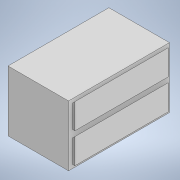
# Autodesk Inventor part: drawer
Saved by Autodesk Inventor 2022 (Build 260153000, 153)
## iProperties
Created: 2022-05-13
Part Number: drawer
Material: Generic
Document SubType Name: Modeling
Designer: compsci
Density: 1 g/cm^3
Appearance: Default
Author: compsci
Autodesk Inventor part; units mm, degrees
ref_plane "YZ Plane" through (0, 0, 0) normal (1, 0, 0) x (0, 1, 0)
ref_plane "XZ Plane" through (0, 0, 0) normal (0, 1, 0) x (-1, 0, 0)
ref_plane "XY Plane" through (0, 0, 0) normal (0, 0, 1) x (1, 0, 0)
sketch "Sketch2" plane through (0, 0, 0) normal (0, 1, 0) x (-1, 0, 0)
  line L0 (-304.8, 508) -> (304.8, 508)
  line L1 (304.8, 508) -> (304.8, -508)
  line L2 (304.8, -508) -> (-304.8, -508)
  line L3 (-304.8, -508) -> (-304.8, 508)
  line L4 (-304.8, 508) -> (304.8, -508) construction
  line L5 (304.8, 508) -> (-304.8, -508) construction
  point P0 (0, 0)
  dimension "d2" = 609.6
  dimension "d3" = 1016
  constraints: 12 end point, 2 midpoint, 2 parallel, 1 horizontal, 1 perpendicular
  measures "d2" distance of L0.start L0.end
  measures "d3" distance of L2.end L0.start
extrude "Extrusion1" add sketch "Sketch2" along normal blind 609.6
sketch "Sketch3" plane through (304.8, 0, 508) normal (1, 0, 0) x (0, 0, -1)
  line L0 (0, 0) -> (1016, 0) projected
  line L1 (1016, 0) -> (1016, 609.6) projected
  line L2 (0, 609.6) -> (1016, 609.6) projected
  line L3 (0, 0) -> (0, 609.6) projected
  line L4 (0, 0) -> (0, 609.6) projected
  line L5 (1016, 0) -> (1016, 609.6) projected
  line L6 (1016, 0) -> (0, 0) projected
  line L7 (0, 304.8) -> (1016, 304.8)
  line L8 (1016, 304.8) -> (1016, 0)
  line L9 (1016, 0) -> (0, 0)
  line L10 (0, 0) -> (0, 304.8)
  line L11 (0, 304.8) -> (1016, 304.8)
  line L12 (1016, 304.8) -> (1016, 609.6)
  line L13 (1016, 609.6) -> (0, 609.6)
  line L14 (0, 609.6) -> (0, 304.8)
  line L15 (977.9, 266.7) -> (38.1, 266.7)
  line L16 (38.1, 266.7) -> (38.1, 38.1)
  line L17 (38.1, 38.1) -> (977.9, 38.1)
  line L18 (977.9, 38.1) -> (977.9, 266.7)
  line L19 (977.9, 342.9) -> (38.1, 342.9)
  line L20 (38.1, 342.9) -> (38.1, 571.5)
  line L21 (38.1, 571.5) -> (977.9, 571.5)
  line L22 (977.9, 571.5) -> (977.9, 342.9)
  point P0 (508, 0)
  dimension "d5" = 38.1
  dimension "d6" = 38.1
  constraints: 32 end point, 8 parallel, 4 perpendicular, 2 horizontal, 1 midpoint, 6 other
  measures "d5" distance between parallel lines of L7 L15
  measures "d6" distance between parallel lines of L11 L19
extrude "Extrusion2" add sketch "Sketch3" along normal blind 25.4 contours L18 L17 L16 L15 | L19 L20 L21 L22
sketch "Sketch4" plane through (304.8, 38.1, 469.9) normal (0, 0, 1) x (1, 0, 0)
  line L0 (0, 304.8) -> (0, 533.4) projected
  line L1 (0, 304.8) -> (25.4, 304.8) projected
  line L2 (25.4, 533.4) -> (25.4, 304.8) projected
  line L3 (0, 533.4) -> (25.4, 533.4) projected
  line L4 (0, 0) -> (0, 228.6) projected
  line L5 (0, 0) -> (25.4, 0) projected
  line L6 (25.4, 228.6) -> (25.4, 0) projected
  line L7 (0, 228.6) -> (25.4, 228.6) projected
  line L8 (25.4, 228.6) -> (25.4, 0) projected
  line L9 (25.4, 228.6) -> (25.4, 254)
  line L10 (0, 228.6) -> (25.4, 228.6) projected
  line L11 (25.4, 254) -> (0, 228.6)
  line L12 (25.4, 533.4) -> (25.4, 304.8) projected
  line L13 (25.4, 533.4) -> (25.4, 558.8)
  line L14 (0, 533.4) -> (25.4, 533.4) projected
  line L15 (25.4, 558.8) -> (0, 533.4)
  point P0 (-304.8, -38.1)
  dimension "d9" = 25.4
  dimension "d10" = 25.4
  constraints: 8 end point, 1 point on line, 1 vertical
  measures "d9" distance of L6.start L9.end
  measures "d10" distance of L2.start L13.end
extrude "Extrusion3" add sketch "Sketch4" against normal up to surface (939.8 mm away) contours L15 L13 L3 | L11 L9 L7
body "Solid1"
